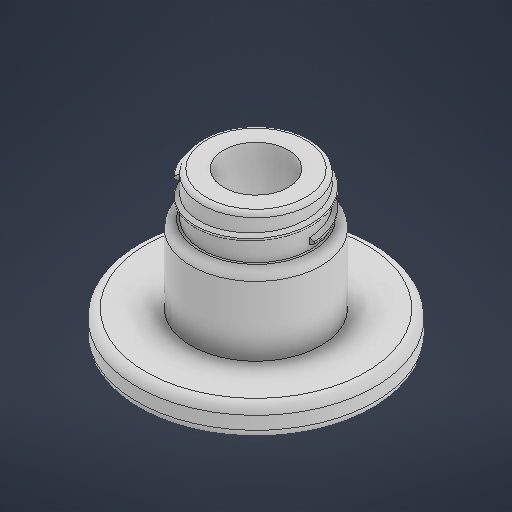
# Autodesk Inventor part: shortspoolv1
Saved by Autodesk Inventor 2027 (Build 310192060, 192F)
## iProperties
Created: 2026-06-22
Part Number: shortspoolv1
Material: Generic
Document SubType Name: Modeling
Designer: beave
Density: 1 g/cm^3
Appearance: Default
Mass: 38.8043 g
Surface Area: 150.775 cm^2
Volume: 38.8043 cm^3
Author: beave
Autodesk Inventor part; units mm, degrees
ref_plane "YZ Plane" through (0, 0, 0) normal (1, 0, 0) x (0, 1, 0)
ref_plane "XZ Plane" through (0, 0, 0) normal (0, 1, 0) x (-1, 0, 0)
ref_plane "XY Plane" through (0, 0, 0) normal (0, 0, 1) x (1, 0, 0)
sketch "Sketch1" plane through (0, 0, 0) normal (0, 1, 0) x (-1, 0, 0)
  circle A0 centre (0, 0) radius 27.5
  dimension "d0" = 55
  constraints: 1 centre point, 1 coincident
  measures "d0" diameter of A0
extrude "Extrusion1" add sketch "Sketch1" along normal blind 7
sketch "Sketch2" plane through (0, 7, 0) normal (0, 1, 0) x (1, 0, 0)
  circle A0 centre (0, 0) radius 15
  dimension "d3" = 30
  constraints: 1 centre point, 1 coincident
  measures "d3" diameter of A0
extrude "Extrusion2" add sketch "Sketch2" along normal blind 18
sketch "Sketch3" plane through (0, 0, 0) normal (0, -1, 0) x (1, 0, 0)
  circle A0 centre (0, 0) radius 27.5 projected
  constraints: 1 coincident
hole "Hole1" at (0, 0, 0) direction (0, 1, 0) diameter 5.8 depth 7 clearance for "Flat Head Machine Screw" size "M5" standard "Ansi Metric M Profile"
sketch "Sketch4" plane through (0, 25, 0) normal (0, 1, 0) x (1, 0, 0)
  circle A0 centre (0, 0) radius 2.9 projected
  circle A1 centre (0, 0) radius 12.5
  dimension "d13" = 25
  constraints: 1 centre point, 1 coincident
  measures "d13" diameter of A1
extrude "Extrusion3" add sketch "Sketch4" along normal blind 10
sketch "Sketch8" plane through (0, 0, 0) normal (0, 0, 1) x (1, 0, 0)
  line L0 (12.5, 73) -> (-12.5, 73) projected
  line L1 (15, 25) -> (-15, 25) projected
  line L2 (12.4688, 27.5) -> (12.4688, 26)
  line L3 (12.4688, 26) -> (13.3929, 26.5335)
  line L4 (13.3929, 26.9665) -> (12.4688, 27.5)
  arc A0 (13.3929, 26.5335) -> (13.3929, 26.9665) centre (13.2679, 26.75) ccw
  circle A1 centre (12.9309, 70.9757) radius 0.75
  point P0 (0, 0)
  point P1 (13.7679, 26.75)
  point P2 (12.4688, 26.75)
  dimension "d30" = 1.5
  dimension "d31" = 60
  dimension "d32" = 0.25
  dimension "d33" = 1
  dimension "d126" = 1.5
  constraints: 6 end point, 2 centre point, 2 point on circle, 2 point on line, 2 tangent, 1 horizontal alignment, 1 midpoint, 1 vertical
  measures "d30" distance of L2.start L2.end
  measures "d31" angle of L3 L4
  measures "d32" radius of A0
  measures "d33" distance from line of L2.end L1
  measures "d126" diameter of A1
coil "Coil1" sketch "Sketch8" operation add axis through (0, -10, 0) along (0, 1, 0) pitch 4 turns 1.625 hand right contours L4 A0 L3 L2
move or copy body "Move Body1" bodies to move or copy 1 copy no translate (0, -0.6, 0)
fillet "Fillet2" radius 1 1 edges at (-12.5, 34.4, 0)
fillet "Fillet3" radius 1 1 edges at (0, -0.6, 2.9)
move or copy body "Move Body2" bodies to move or copy 1 copy no translate (0, -4.58, 0)
sketch "Sketch24" plane through (0, 29.82, 0) normal (0, 1, 0) x (1, 0, 0)
  circle A0 centre (0, 0) radius 12.5 projected
  constraints: 1 coincident
hole "Hole3" at (0, 29.82, 0) direction (0, -1, 0) diameter 15 depth 28
sketch "Sketch27" plane through (0, 1.82, 0) normal (0, 1, 0) x (1, 0, 0)
  point P0 (0, 0)
sketch "Sketch30" plane through (0, 1.82, 0) normal (0, 1, 0) x (1, 0, 0)
  circle A0 centre (0, 0) radius 27.5 projected
  constraints: 1 coincident
hole "Hole6" at (0, 1.82, 0) direction (0, 1, 0) diameter 5.8 depth 3 tip angle 118 clearance for "Hex Head Machine Screw" size "M5" standard "Ansi Metric M Profile"
fillet "Fillet5" radius 2 2 edges at (27.5, 1.82, 0) (27.5, -5.18, 0)
fillet "Fillet6" radius 2 1 edges at (-15, 19.82, 0)
body "Solid1"
